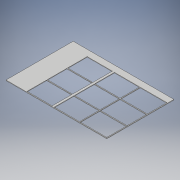
# Autodesk Inventor part: Test_Panel
Saved by Autodesk Inventor 2019.4 (Build 234330000, 330)
## iProperties
Created: 2020-02-07
Part Number: Test_Panel
Material: Generic
Document SubType Name: Modeling
Designer: Jorian Bruslind
Density: 1 g/cm^3
Appearance: Default
Author: Jorian Bruslind
Autodesk Inventor part; units mm, degrees
ref_plane "YZ Plane" through (0, 0, 0) normal (1, 0, 0) x (0, 1, 0)
ref_plane "XZ Plane" through (0, 0, 0) normal (0, 1, 0) x (-1, 0, 0)
ref_plane "XY Plane" through (0, 0, 0) normal (0, 0, 1) x (1, 0, 0)
sketch "Sketch1" plane through (0, 0, 0) normal (0, 1, 0) x (-1, 0, 0)
  line L0 (0, 0) -> (-1828.8, 0)
  line L1 (-1828.8, 0) -> (-1828.8, -1219.2)
  line L2 (-1828.8, -1219.2) -> (0, -1219.2)
  line L3 (0, -1219.2) -> (0, 0)
  line L4 (-1828.8, 0) -> (-1828.8, -12.7)
  line L5 (-1828.8, -12.7) -> (-1816.1, -12.7)
  line L6 (-1816.1, -12.7) -> (-1333.5, -12.7)
  line L7 (-1333.5, -12.7) -> (-1333.5, -368.3)
  line L8 (-1333.5, -368.3) -> (-1816.1, -368.3)
  line L9 (-1816.1, -368.3) -> (-1816.1, -12.7)
  line L10 (-1333.5, -381) -> (-1333.5, -736.6)
  line L11 (-1333.5, -736.6) -> (-1816.1, -736.6)
  line L12 (-1816.1, -736.6) -> (-1816.1, -381)
  line L13 (-1816.1, -381) -> (-1333.5, -381)
  line L14 (-1333.5, -749.3) -> (-1333.5, -1104.9)
  line L15 (-1333.5, -1104.9) -> (-1816.1, -1104.9)
  line L16 (-1816.1, -1104.9) -> (-1816.1, -749.3)
  line L17 (-1816.1, -749.3) -> (-1333.5, -749.3)
  line L18 (-1333.5, -12.7) -> (-1320.8, -12.7)
  line L19 (-1320.8, -12.7) -> (-863.6, -12.7)
  line L20 (-863.6, -12.7) -> (-863.6, -368.3)
  line L21 (-863.6, -368.3) -> (-1320.8, -368.3)
  line L22 (-1320.8, -368.3) -> (-1320.8, -12.7)
  line L23 (-863.6, -736.6) -> (-1320.8, -736.6)
  line L24 (-1320.8, -736.6) -> (-1320.8, -381)
  line L25 (-1320.8, -381) -> (-863.6, -381)
  line L26 (-863.6, -381) -> (-863.6, -736.6)
  line L27 (-863.6, -1104.9) -> (-1320.8, -1104.9)
  line L28 (-1320.8, -1104.9) -> (-1320.8, -749.3)
  line L29 (-1320.8, -749.3) -> (-863.6, -749.3)
  line L30 (-863.6, -749.3) -> (-863.6, -1104.9)
  line L31 (-368.3, -368.3) -> (-825.5, -368.3)
  line L32 (-825.5, -368.3) -> (-825.5, -12.7)
  line L33 (-825.5, -12.7) -> (-368.3, -12.7)
  line L34 (-368.3, -12.7) -> (-368.3, -368.3)
  line L35 (-368.3, -736.6) -> (-825.5, -736.6)
  line L36 (-825.5, -736.6) -> (-825.5, -381)
  line L37 (-825.5, -381) -> (-368.3, -381)
  line L38 (-368.3, -381) -> (-368.3, -736.6)
  line L39 (-368.3, -1104.9) -> (-825.5, -1104.9)
  line L40 (-825.5, -1104.9) -> (-825.5, -749.3)
  line L41 (-825.5, -749.3) -> (-368.3, -749.3)
  line L42 (-368.3, -749.3) -> (-368.3, -1104.9)
  dimension "d0" = 1828.8
  dimension "d1" = 1219.2
  dimension "d2" = 12.7
  dimension "d3" = 12.7
  dimension "d4" = 482.6
  dimension "d5" = 355.6
  dimension "d8" = 368.3
  dimension "d13" = 12.7
  dimension "d14" = 457.2
  dimension "d15" = 355.6
  dimension "d18" = 368.3
  dimension "d21" = 495.3
  constraints: 86 end point, 6 horizontal, 6 parallel, 3 perpendicular, 2 vertical, 1 point on line, 56 other
  measures "d0" distance of L2.end L1.end
  measures "d1" distance of L1.end L0.end
  measures "d2" distance of L0.end L4.end
  measures "d3" distance of L4.end L5.end
  measures "d4" distance of L7.end L8.end
  measures "d5" distance of L6.end L7.end
  measures "d8" distance of L6.end L10.start
  measures "d13" distance of L6.end L18.end
  measures "d14" distance of L20.end L21.end
  measures "d15" distance of L19.end L20.end
  measures "d18" distance of L20.end L23.start
  measures "d21" distance of L20.end L31.start
extrude "Extrusion1" add sketch "Sketch1" along normal blind 10
body "Solid1"
